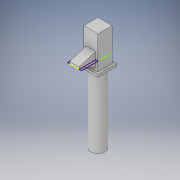
# Autodesk Inventor part: pin
Saved by Autodesk Inventor 2019 (Build 230136000, 136)
## iProperties
Created: 2020-07-23
Part Number: pin
Material: Generic
Document SubType Name: Modeling
Designer: lukad
Density: 1 g/cm^3
Appearance: Default
Author: lukad
Autodesk Inventor part; units mm, degrees
ref_plane "YZ Plane" through (0, 0, 0) normal (1, 0, 0) x (0, 1, 0)
ref_plane "XZ Plane" through (0, 0, 0) normal (0, 1, 0) x (-1, 0, 0)
ref_plane "XY Plane" through (0, 0, 0) normal (0, 0, 1) x (1, 0, 0)
sketch "Sketch1" plane through (0, 0, 0) normal (0, 1, 0) x (-1, 0, 0)
  circle A0 centre (1.1561, 1.8072) radius 3
  line L0 (4.1561, 4.8072) -> (-1.8439, 4.8072)
  line L1 (-1.8439, 4.8072) -> (-1.8439, -1.1928)
  line L2 (-1.8439, -1.1928) -> (4.1561, -1.1928)
  line L3 (4.1561, -1.1928) -> (4.1561, 4.8072)
  point P0 (0, 0)
  dimension "d0" = 6
  constraints: 8 end point, 2 parallel, 1 centre point, 1 horizontal, 1 perpendicular
  measures "d0" diameter of A0
extrude "Extrusion1" add sketch "Sketch1" along normal blind 10
extrude "Extrusion2" add sketch "Sketch1" against normal blind 20 contours A0
sketch "Sketch2" plane through (-4.1561, 10, 4.8072) normal (0, 0, 1) x (1, 0, 0)
  line L0 (0, -10) -> (0, 0) projected
  line L1 (6, -10) -> (0, -10)
  line L2 (0, -10) -> (0, -7)
  line L3 (0, -7) -> (6, -7)
  line L4 (6, -7) -> (6, -10)
  line L5 (0, 0) -> (6, 0) projected
  line L6 (0, -30) -> (6, -30) projected
  line L7 (3, -10) -> (6, -10) projected
  point P0 (4.1561, -10)
  dimension "d5" = 3
  dimension "d6" = 6
  dimension "d7" = 30
  dimension "d13" = 0
  constraints: 8 end point, 2 parallel, 1 collinear, 1 horizontal, 1 perpendicular, 1 point on line
  measures "d5" distance between parallel lines of L3 L1
  measures "d6" distance between parallel lines of L0 L4
  measures "d7" distance between parallel lines of L5 L6
  measures "d13" distance between parallel lines of L7 L1
extrude "Extrusion3" add sketch "Sketch2" along normal blind 7
sketch "Sketch3" plane through (-4.1561, 0, -1.1928) normal (-1, 0, 0) x (0, 0, 1)
  line L0 (6, 3) -> (13, 3) projected
  line L1 (13, 3) -> (13, 0) projected
  arc A0 (9.5, 3) -> (13, 1.5) centre (12.6357, 5.4834) ccw
  point P0 (1.1928, 0)
  dimension "d10" = 4
  constraints: 2 midpoint, 2 point on circle, 1 centre point
  measures "d10" radius of A0
extrude "Extrusion4" [suppressed]
fillet "Fillet1" [suppressed]
fillet "Fillet2" [suppressed]
fillet "Fillet3" [suppressed]
sketch "Sketch4" plane through (1.8439, 0, -1.1928) normal (1, 0, 0) x (0, 0, -1)
  line L0 (-6, 3) -> (-13, 3) projected
  line L1 (-6, 3) -> (-13, 0.7757)
  line L2 (-13, 3) -> (-13, 0) projected
  line L3 (-13, 0.7757) -> (-13, 3)
  line L4 (-6, 3) -> (-13, 3) projected
  line L5 (-13, 3) -> (-6, 3)
  point P0 (-1.1928, 0)
  constraints: 6 end point, 1 collinear, 1 vertical
extrude "Extrusion5" cut sketch "Sketch4" against normal blind 10
sketch "Sketch5" plane through (0, 0, 0) normal (0, -1, 0) x (1, 0, 0)
  line L0 (-4.1561, 4.8072) -> (1.8439, 4.8072) projected
  line L1 (-4.1561, 11.8072) -> (1.8439, 11.8072) projected
  line L2 (1.8439, 4.8072) -> (0.8439, 4.8072)
  line L3 (0.8439, 4.8072) -> (0.8439, 11.8072)
  line L4 (0.8439, 11.8072) -> (1.8439, 11.8072)
  line L5 (1.8439, 11.8072) -> (1.8439, 4.8072)
  line L6 (-3.1561, 4.8072) -> (-4.1561, 4.8072)
  line L7 (-4.1561, 4.8072) -> (-4.1561, 11.8072)
  line L8 (-4.1561, 11.8072) -> (-3.1561, 11.8072)
  line L9 (-3.1561, 11.8072) -> (-3.1561, 4.8072)
  line L10 (-3.1561, 10.3072) -> (0.8439, 10.3072)
  point P0 (0, 0)
  dimension "d19" = 6
  dimension "d20" = 1
  dimension "d21" = 1
  dimension "d28" = 1.5
  constraints: 18 end point, 5 parallel, 4 point on line, 3 perpendicular, 2 horizontal
  measures "d19" distance of L1.start L1.end
  measures "d20" distance between parallel lines of L5 L3
  measures "d21" distance between parallel lines of L7 L9
  measures "d28" distance between parallel lines of L1 L10
extrude "Extrusion6" cut sketch "Sketch5" against normal blind 10 contours L3 L1 L5 L0
extrude "Extrusion7" cut sketch "Sketch5" against normal blind 10 contours L7 L1 L9 L0
extrude "Extrusion8" add sketch "Sketch1" against normal blind 5 contours L3 L2 A0 | A0 L0 L3 | A0 L1 L0 | L2 L1 A0
sketch "Sketch6" plane through (0.8439, 0, 11.8072) normal (1, 0, 0) x (0, 0, -1)
  point P0 (11.8072, 0)
sketch "Sketch7" plane through (0.8439, 0, 11.8072) normal (1, 0, 0) x (0, 0, -1)
  point P0 (11.8072, 0)
extrude "Extrusion9" add sketch "Sketch5" along normal blind 3 contours L9 L10 L3 L0
sketch "Sketch9" plane through (0.8439, 0, 11.8072) normal (1, 0, 0) x (0, 0, -1)
  line L0 (7, -3) -> (1.5, 0)
  line L1 (1.5, 0) -> (7, 0)
  line L2 (7, -3) -> (7, 3) projected
  line L3 (1.5, 0) -> (1.5, -3) projected
  line L4 (1.5, -3) -> (7, -3)
  point P0 (11.8072, 0)
  constraints: 6 end point, 1 horizontal, 1 midpoint
extrude "Extrusion10" cut sketch "Sketch9" against normal blind 5 contours L4 L3 L0
sketch "Sketch10" plane through (0, -5, 0) normal (0, -1, 0) x (1, 0, 0)
  line L0 (2.8439, 5.8072) -> (-5.1561, 5.8072)
  line L1 (-5.1561, 5.8072) -> (-5.1561, -2.1928)
  line L2 (-5.1561, -2.1928) -> (2.8439, -2.1928)
  line L3 (2.8439, -2.1928) -> (2.8439, 5.8072)
  line L4 (1.8439, 1.8072) -> (1.8439, 4.8072) projected
  line L5 (-1.1561, -1.1928) -> (1.8439, -1.1928) projected
  line L6 (1.8439, 4.8072) -> (-1.1561, 4.8072) projected
  line L7 (-4.1561, 4.8072) -> (-4.1561, 1.8072) projected
  point P0 (0, 0)
  dimension "d33" = 1
  dimension "d34" = 1
  dimension "d35" = 1
  dimension "d36" = 1
  constraints: 8 end point, 2 parallel, 1 horizontal, 1 perpendicular
  measures "d33" distance between parallel lines of L4 L3
  measures "d34" distance between parallel lines of L5 L2
  measures "d35" distance between parallel lines of L0 L6
  measures "d36" distance between parallel lines of L1 L7
extrude "Extrusion11" add sketch "Sketch10" against normal blind 1
sketch "Sketch11" plane through (-1.1561, -20, 1.8072) normal (0, -1, 0) x (1, 0, 0)
  circle A0 centre (0, 0) radius 3
  circle A1 centre (0, 0) radius 3 projected
  point P0 (1.1561, -1.8072)
  dimension "d39" = 6
  constraints: 1 centre point, 1 concentric
  measures "d39" diameter of A0
extrude "Extrusion12" add sketch "Sketch11" along normal blind 15
body "Solid1"
